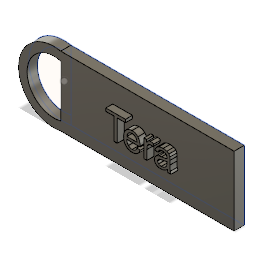
铭牌 (Autodesk Fusion 360 design; units mm, degrees)
Autodesk Fusion 360 part; units mm, degrees
sketch "草图11" plane through (0, 0, 0) normal (0, 0, 1) x (1, 0, 0)
  line L0 (-50, 25) -> (0, 25)
  line L1 (0, 25) -> (0, 5)
  line L2 (0, 5) -> (-50, 5)
  line L3 (-50, 5) -> (-50, 25)
  arc A0 (-50, 25) -> (-50, 5) centre (-51.9859, 15) ccw
  arc A1 (-50, 22.4346) -> (-50, 7.5654) centre (-51.9859, 15) ccw
extrude "拉伸2" add sketch "草图11" along normal blind 3 contours L3 A0 A1 makes body 1
extrude "拉伸1" add sketch "草图11" along normal blind 3 separate body contours L0 L1 L2 L3 makes body 2
sketch "草图12" plane through (0, 0, 3) normal (0, 0, 1) x (1, 0, 0)
  line L0 (-50, 5) -> (0, 5)
  line L1 (0, 5) -> (0, 25)
  line L2 (0, 25) -> (-50, 25)
  line L3 (-50, 25) -> (-50, 5)
  line L4 (-35, 12) -> (-16.2061, 12) construction
  line L5 (-16.2061, 12) -> (-16.2061, 22) construction
  line L6 (-16.2061, 22) -> (-35, 22) construction
  line L7 (-35, 22) -> (-35, 12) construction
  text T0 "Tera" font "Arial" height 10 align ink ink in box 0 x 0 at (-35, 12) x (1, 0) y (0, 1) spacing 1 kerned height is em
extrude "拉伸3" add sketch "草图12" along normal blind 2 text T0 bodies 2
combine "合并4" operation add target body 1 tool bodies 2
